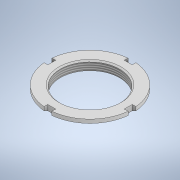
# Autodesk Inventor part: 76. Гайка первичного вала
Saved by Autodesk Inventor 2021 (Build 250183000, 183)
## iProperties
Created: 2021-03-15
Part Number: 76. Гайка первичного вала
Material: Типовые
Document SubType Name: Modeling
Designer: Данил
Density: 1 g/cm^3
Appearance: По умолчанию
Author: Данил
Autodesk Inventor part; units mm, degrees
ref_plane "YZ Plane" through (0, 0, 0) normal (1, 0, 0) x (0, 1, 0)
ref_plane "XZ Plane" through (0, 0, 0) normal (0, 1, 0) x (-1, 0, 0)
ref_plane "XY Plane" through (0, 0, 0) normal (0, 0, 1) x (1, 0, 0)
sketch "Эскиз1" plane through (0, 0, 0) normal (0, 0, 1) x (1, 0, 0)
  line L0 (0, 3.5) -> (0, -3.5)
  line L1 (0, -3.5) -> (23, -3.5) construction
  line L2 (23, -3.5) -> (22.5, -3.2113)
  line L3 (22.5, -3.2113) -> (22.5, 2.5)
  line L4 (23.5, 3.5) -> (32, 3.5)
  line L5 (32, 3.5) -> (32, 0.6968)
  line L6 (32, 0.6968) -> (23, -3.5)
  line L7 (22.5, 2.5) -> (23.5, 3.5)
  point P0 (0, 0)
  point P1 (0, 0)
  point P2 (22.5, 3.5)
  dimension "d0" = 7
  dimension "d1" = 46
  dimension "d2" = 45
  dimension "d3" = 25
  dimension "d5" = 64
  dimension "d6" = 1
  dimension "d7" = 45
  dimension "d8" = 60
  constraints: 16 end point, 2 perpendicular, 2 point on line, 2 vertical, 1 coincident, 1 horizontal, 1 horizontal alignment, 1 midpoint
  measures "d0" distance of L0.start L0.end
  measures "d1" diameter of L1.end L0
  measures "d2" diameter of L3 L0
  measures "d3" angle of L1 L6
  measures "d5" diameter of L5 L0
  measures "d6" distance of L3.end point (22.5, 3.5)
  measures "d7" angle of L3 L7
  measures "d8" angle of L0 L2
revolve "Вращение1" add sketch "Эскиз1" angle 360 about axis through (0, 3.5, 0) along (0, -1, 0)
sketch "Эскиз2" plane through (0, 3.5, 0) normal (0, 1, 0) x (1, 0, 0)
  line L0 (-3, 32) -> (3, 32)
  line L1 (3, 32) -> (3, 29)
  line L2 (3, 29) -> (-3, 29)
  line L3 (-3, 29) -> (-3, 32)
  circle A0 centre (0, 0) radius 32 projected
  point P0 (0, 0)
  point P1 (0, 29)
  point P2 (3, 31.8591)
  point P3 (-3, 31.8591)
  dimension "d10" = 6
  dimension "d11" = 3
  constraints: 8 end point, 2 parallel, 1 horizontal, 1 midpoint, 1 perpendicular, 1 tangent, 1 vertical alignment
  measures "d10" distance of L0.start L0.end
  measures "d11" distance of L0.end L1.end
extrude "Выдавливание1" cut sketch "Эскиз2" against normal through all contours A0 L1 L2 L3 picked at (0, 30)
pattern_circular "Круговой массив1" count 4 over 360 about axis through (0, -0.3557, 0) along (0, -1, 0) of "Выдавливание1"
thread "Резьба1" size "M45x1.5" class "6H" standard "ISO Metric profile" length 20
